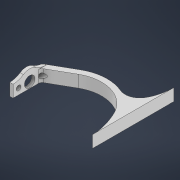
# Autodesk Inventor part: Antenna_table_holder
Saved by Autodesk Inventor 2022 (Build 260153000, 153)
## iProperties
Created: 2022-04-09
Part Number: Antenna_table_holder
Material: Generic
Document SubType Name: Modeling
Designer: dvorakj
Density: 1 g/cm^3
Appearance: Default
Author: dvorakj
Autodesk Inventor part; units mm, degrees
ref_plane "YZ Plane" through (0, 0, 0) normal (1, 0, 0) x (0, 1, 0)
ref_plane "XZ Plane" through (0, 0, 0) normal (0, 1, 0) x (-1, 0, 0)
ref_plane "XY Plane" through (0, 0, 0) normal (0, 0, 1) x (1, 0, 0)
sketch "Sketch1" plane through (0, 0, 0) normal (0, 1, 0) x (-1, 0, 0)
  line L0 (0, 0) -> (0, -5)
  arc A0 (0, -5) -> (0.4476, -10.3333) centre (32, -5) ccw
  arc A1 (0.4476, -10.3333) -> (30.0699, -24.3767) centre (20.1678, -7) ccw
  line L1 (30.0699, -24.3767) -> (42.0669, -17.5402)
  line L2 (44.8693, -17) -> (44.8693, -20)
  arc A2 (44.8693, -20) -> (42.8889, -20.5247) centre (44.8693, -24) ccw
  line L3 (42.8889, -20.5247) -> (31.5553, -26.9832)
  arc A3 (11.1401, -28.1542) -> (31.5553, -26.9832) centre (20.1678, -7) ccw
  arc A4 (11.1401, -28.1542) -> (0, -35.5122) centre (8, -35.5122) ccw
  line L4 (0, -35.5122) -> (0, -44)
  line L5 (0, 0) -> (-2, 0)
  line L6 (-2, 0) -> (-2, -44)
  line L7 (-2, -44) -> (0, -44)
  line L8 (43.0767, -15.8025) -> (43.0767, -2)
  line L9 (43.0767, -2) -> (44.8693, -2)
  line L10 (44.8693, -2) -> (44.8693, -17)
  arc A5 (42.0669, -17.5402) -> (43.0767, -15.8025) centre (41.0767, -15.8025) ccw
  line L11 (-2, 0) -> (-2, -3.5632) construction
  line L12 (-2, -3.5632) -> (-1.4448, -6.2034) construction
  line L13 (-1.4448, -6.2034) -> (0.0001, -11.3997) construction
  line L14 (0.0001, -11.3997) -> (2.2909, -15.9674) construction
  spline S0 degree 4 poles (-2, 0) (-2, -3.5632) (-1.4448, -6.2034) (0.0001, -11.3997) (2.2909, -15.9674) knots 1 1 1 1 1 2 2 2 2 2
  line L15 (-2, -44) -> (-2, -40.2379) construction
  spline S1 degree 3 poles (-2, -44) (-2, -40.2379) (-1.2855, -35.1022) (1.3006, -31.1398) knots 1 1 1 1 1.689473 1.689473 1.689473 1.689473
  line L16 (-2, -40.2379) -> (-1.2855, -35.1022) construction
  line L17 (-1.2855, -35.1022) -> (1.3006, -31.1398) construction
  point P0 (41.4036, -17.9182)
  point P1 (6.6915, -28.5942)
  point P2 (6.6915, -28.5942)
  point P3 (2.2892, -15.964)
  dimension "d0" = 3
  dimension "d1" = 44.8693
  dimension "d2" = 4
  dimension "d5" = 32
  dimension "d6" = 20
  dimension "d7" = 5
  dimension "d8" = 7
  dimension "d10" = 17
  dimension "d11" = 8
  dimension "d12" = 44
  dimension "d13" = 2
  dimension "d16" = 2
  dimension "d17" = 15
  constraints: 22 end point, 13 point on circle, 9 tangent, 6 centre point, 5 vertical, 4 perpendicular, 2 coincident, 2 parallel, 1 horizontal, 1 line through centre, 1 point on line, 1 vertical alignment, 10 other
  measures "d0" radial gap between concentric circles of A3 A1
  measures "d1" distance between parallel lines of L0 L2
  measures "d2" radius of A2
  measures "d5" radius of A0
  measures "d6" radius of A1
  measures "d7" distance of L0.start L0.end
  measures "d8" vertical distance of L0.start A1.centre
  measures "d10" vertical distance of L0.start L2.start
  measures "d11" radius of A4
  measures "d12" distance of L5.end L6.end
  measures "d13" distance from line of L0.start L6
  measures "d16" radius of A5
  measures "d17" vertical distance of L2.start L8.end
extrude "Extrusion1" add sketch "Sketch1" along normal blind 6.5 contours S0 A1 L1 A5 L8 L9 L10 L2 A2 L3 A3 A4 S1 L6
sketch "Sketch2" plane through (-44.8693, 0, -20) normal (-1, 0, 0) x (0, 0, 1)
  line L0 (0, 0) -> (18, 0) projected
  line L1 (18, 0) -> (18, 6.5) projected
  line L2 (0, 6.5) -> (18, 6.5) projected
  line L3 (0, 0) -> (0, 6.5) projected
  circle A0 centre (15, 3.25) radius 1.3
  circle A1 centre (3, 3.25) radius 1.3
  line L4 (0, 0) -> (18, 0) projected
  line L5 (18, 0) -> (18, 6.5) projected
  circle A2 centre (9, 3.25) radius 2.85
  point P0 (20, 0)
  point P1 (9, 0)
  point P2 (18, 3.25)
  dimension "d18" = 2.6
  dimension "d19" = 2.6
  dimension "d20" = 12
  dimension "d21" = 6
  dimension "d22" = 5.7
  constraints: 3 centre point, 2 horizontal alignment, 2 midpoint
  measures "d18" diameter of A0
  measures "d19" diameter of A1
  measures "d20" distance of A1.centre A0.centre
  measures "d21" horizontal distance of point (9, 0) A0.centre
  measures "d22" diameter of A2
extrude "Extrusion2" cut sketch "Sketch2" against normal blind 6.5 contours A0 | A1 | A2
sketch "Sketch3" plane through (-44.8693, 0, -20) normal (-1, 0, 0) x (0, 0, 1)
  circle A0 centre (3, 3.25) radius 1.3 projected
  circle A1 centre (9, 3.25) radius 2.85 projected
  circle A2 centre (15, 3.25) radius 1.3 projected
  line L0 (0, 0) -> (18, 0) projected
  line L1 (18, 0) -> (18, 6.5) projected
  line L2 (0, 6.5) -> (18, 6.5) projected
  line L3 (0, 0) -> (0, 6.5) projected
  circle A3 centre (9, 3.25) radius 6
  line L4 (0, 6.5) -> (18, 6.5) projected
  line L5 (18, 6.5) -> (0, 6.5)
  point P0 (20, 0)
  point P1 (14.0436, 6.5)
  point P2 (3.9564, 6.5)
  dimension "d25" = 12
  constraints: 2 end point, 1 centre point, 1 coincident, 1 collinear
  measures "d25" diameter of A3
extrude "Extrusion3" add sketch "Sketch3" against normal up to surface (1.7926 mm away) contours A3 L2
fillet "Fillet1" radius 10 2 edges at (-43.973, 6.5, -5.9564) (-43.973, 6.5, -16.0436)
fillet "Fillet2" radius 2 1 edges at (-44.8693, 3.25, -20)
equation "\"d19\" = d18"
equation "\"d21\" = 0.5 * d20"
body "Solid1"
